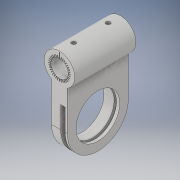
# Autodesk Inventor part: cam_holder_wrist_part
Saved by Autodesk Inventor 2019 (Build 230136000, 136)
## iProperties
Created: 2024-08-06
Part Number: cam_holder_wrist_part
Material: Generisch
Document SubType Name: Modeling
Designer: nic
Density: 1 g/cm^3
Appearance: Vorgabe
Author: nic
Autodesk Inventor part; units mm, degrees
ref_plane "YZ Plane" through (0, 0, 0) normal (1, 0, 0) x (0, 1, 0)
ref_plane "XY Plane" through (0, 0, 0) normal (0, 0, 1) x (1, 0, 0)
sketch "Skizze1" plane through (0, 0, 0) normal (1, 0, 0) x (0, 1, 0)
  line L0 (0, 0) -> (0, 35) construction
  circle A0 centre (0, 35) radius 35
  circle A1 centre (0, 35) radius 25.05
  dimension "d0" = 35
  dimension "d1" = 50.1
  constraints: 2 coincident, 2 end point, 1 centre point, 1 vertical, 1 vertical alignment, 2 other
  measures "d0" distance of L0.start L0.end
  measures "d1" diameter of A1
extrude "Extrusion1" add sketch "Skizze1" along normal blind 18
sketch "Skizze2" plane through (0, 0, 0) normal (0, 0, 1) x (1, 0, 0)
  line L0 (18, -35) -> (18, 35) construction
  line L1 (0, 35) -> (0, -35) construction
  line L2 (0, 35) -> (18, 35) projected
  line L3 (9, 35) -> (9, 60) construction
  circle A0 centre (9, 60) radius 10.05
  circle A1 centre (9, 60) radius 17.5
  point P0 (0, 0)
  dimension "d5" = 25
  dimension "d6" = 20.1
  dimension "d7" = 35
  constraints: 2 centre point, 2 coincident, 2 end point, 1 midpoint, 1 vertical
  measures "d5" distance of L3.start L3.end
  measures "d6" diameter of A0
  measures "d7" diameter of A1
extrude "Extrusion2" add sketch "Skizze2" along normal blind 70
sketch "Skizze3" plane through (0, 0, 0) normal (0, 0, 1) x (1, 0, 0)
  line L0 (18, -35) -> (18, 35) construction
  line L1 (0, 35) -> (0, -35) construction
  circle A0 centre (9, 60) radius 17.5 construction
  line L2 (18, -35) -> (18, 35) projected
  line L3 (18, 0) -> (0, 0)
  line L4 (0, 0) -> (0, 44.9917)
  line L5 (18, 44.9917) -> (18, 0)
  arc A1 (0, 44.9917) -> (18, 44.9917) centre (9, 60) ccw
  point P0 (0, 0)
  constraints: 6 end point, 2 point on circle, 1 centre point, 1 coincident, 1 horizontal, 1 midpoint, 1 parallel, 1 perpendicular, 2 other
extrude "Extrusion3" add sketch "Skizze3" along normal blind 70
sketch "Skizze4" plane through (0, 0, 0) normal (-1, 0, 0) x (0, 0, 1)
  line L0 (9.95, 0) -> (60.05, 0) projected
  circle A0 centre (35, 0) radius 25.05
  point P0 (0, 0)
  constraints: 1 centre point, 1 midpoint
extrude "Extrusion4" cut sketch "Skizze4" against normal through all
ref_plane "Arbeitsebene1" through (13, 0, 0) normal (1, 0, 0) x (0, 0, -1)
sketch "Skizze5" plane through (13, 0, 0) normal (1, 0, 0) x (0, 0, -1)
  circle A0 centre (-35, 0) radius 25.05 construction
  arc A1 (-70, 0) -> (0, 0) centre (-35, 0) ccw construction
  line L0 (0, 44.9917) -> (0, 0) construction
  line L1 (-70, 44.9917) -> (0, 44.9917) construction
  line L2 (-70, 0) -> (-70, 44.9917) construction
  circle A2 centre (-35, 0) radius 25.05
  arc A3 (-59.4438, 25.05) -> (-10.5562, 25.05) centre (-35, 0) ccw
  line L3 (-70, 0) -> (-70, 44.9917) projected
  line L4 (-70, 25.05) -> (0, 25.05)
  line L5 (0, 25.05) -> (0, 0)
  line L6 (-70, 0) -> (-70, 25.05)
  constraints: 6 end point, 4 point on circle, 3 point on line, 2 centre point, 2 coincident, 1 horizontal, 1 parallel, 1 perpendicular
extrude "Extrusion5" cut sketch "Skizze5" against normal blind 1.325 and the other way blind 1.325
sketch "Skizze6" plane through (13, 0, 0) normal (1, 0, 0) x (0, 0, -1)
  circle A0 centre (-35, 0) radius 25.05 construction
  arc A1 (-70, 0) -> (0, 0) centre (-35, 0) ccw construction
  line L0 (0, 44.9917) -> (0, 0) construction
  line L1 (-70, 44.9917) -> (0, 44.9917) construction
  line L2 (-70, 0) -> (-70, 44.9917) construction
  arc A2 (-70, 0) -> (0, 0) centre (-35, 0) ccw projected
  line L3 (-70, 25.05) -> (-70, 0) projected
  line L4 (0, 0) -> (0, 25.05) projected
  line L5 (-70, 25.05) -> (-35, 25.05) projected
  line L6 (-35, 25.05) -> (0, 25.05) projected
  line L7 (-65, 39.9917) -> (-5, 39.9917)
  line L8 (-5, 39.9917) -> (-5, 0)
  arc A3 (-65, 0) -> (-5, 0) centre (-35, 0) ccw
  line L9 (-65, 0) -> (-65, 39.9917)
  line L10 (-65, 25.05) -> (-5, 25.05)
  dimension "d19" = 5
  constraints: 8 end point, 4 point on line, 2 point on circle, 1 centre point, 1 vertical alignment, 3 other
  measures "d19" distance between parallel lines of L2 L9
extrude "Extrusion6" cut sketch "Skizze6" against normal blind 2.5 and the other way blind 2.5 contours L3 L5 L9 A3 L8 L6 L4 A2
ref_plane "Arbeitsebene2" through (0, 78, 0) normal (0, 1, 0) x (-1, 0, 0)
sketch "Skizze7" plane through (0, 78, 0) normal (0, 1, 0) x (-1, 0, 0)
  line L0 (-19.05, 70) -> (1.05, 70) projected
  line L1 (-9, 70) -> (-9, 0)
  point P0 (0, 0)
  point P1 (-9, 53.6501)
  point P2 (-9, 14.2598)
  constraints: 2 end point, 2 point on line, 1 midpoint, 1 vertical
hole "Bohrung1" at (9, 78, 53.6501) at (9, 78, 14.2598) direction (0, -1, 0) diameter 3.8 depth 10 tip angle 118 counterbore diameter 5 counterbore depth 2
sketch "Skizze8" plane through (0, 0, 70) normal (0, 0, 1) x (1, 0, 0)
  circle A0 centre (9, 60) radius 10.05 construction
  arc A1 (18, 44.9917) -> (0, 44.9917) centre (9, 60) ccw construction
  line L0 (8.75, 67.55) -> (9.25, 67.55)
  line L1 (9.25, 67.55) -> (9.25, 72.55)
  line L2 (9.25, 72.55) -> (8.75, 72.55)
  line L3 (8.75, 72.55) -> (8.75, 67.55)
  line L4 (8.75, 67.55) -> (9.25, 72.55) construction
  line L5 (9.25, 67.55) -> (8.75, 72.55) construction
  line L6 (7.4428, 67.3919) -> (7.9352, 67.4787)
  line L7 (7.9352, 67.4787) -> (7.0669, 72.4027)
  line L8 (7.0669, 72.4027) -> (6.5745, 72.3159)
  line L9 (6.5745, 72.3159) -> (7.4428, 67.3919)
  line L10 (7.4428, 67.3919) -> (7.0669, 72.4027) construction
  line L11 (7.9352, 67.4787) -> (6.5745, 72.3159) construction
  line L12 (6.1828, 67.0092) -> (6.6527, 67.1802)
  line L13 (6.6527, 67.1802) -> (4.9426, 71.8786)
  line L14 (4.9426, 71.8786) -> (4.4727, 71.7076)
  line L15 (4.4727, 71.7076) -> (6.1828, 67.0092)
  line L16 (6.1828, 67.0092) -> (4.9426, 71.8786) construction
  line L17 (6.6527, 67.1802) -> (4.4727, 71.7076) construction
  line L18 (5.0085, 66.4135) -> (5.4415, 66.6635)
  line L19 (5.4415, 66.6635) -> (2.9415, 70.9936)
  line L20 (2.9415, 70.9936) -> (2.5085, 70.7436)
  line L21 (2.5085, 70.7436) -> (5.0085, 66.4135)
  line L22 (5.0085, 66.4135) -> (2.9415, 70.9936) construction
  line L23 (5.4415, 66.6635) -> (2.5085, 70.7436) construction
  line L24 (3.9554, 65.6229) -> (4.3385, 65.9443)
  line L25 (4.3385, 65.9443) -> (1.1245, 69.7746)
  line L26 (1.1245, 69.7746) -> (0.7415, 69.4532)
  line L27 (0.7415, 69.4532) -> (3.9554, 65.6229)
  line L28 (3.9554, 65.6229) -> (1.1245, 69.7746) construction
  line L29 (4.3385, 65.9443) -> (0.7415, 69.4532) construction
  line L30 (3.0557, 64.6615) -> (3.3771, 65.0446)
  line L31 (3.3771, 65.0446) -> (-0.4532, 68.2585)
  line L32 (-0.4532, 68.2585) -> (-0.7746, 67.8755)
  line L33 (-0.7746, 67.8755) -> (3.0557, 64.6615)
  line L34 (3.0557, 64.6615) -> (-0.4532, 68.2585) construction
  line L35 (3.3771, 65.0446) -> (-0.7746, 67.8755) construction
  line L36 (2.3365, 63.5585) -> (2.5865, 63.9915)
  line L37 (2.5865, 63.9915) -> (-1.7436, 66.4915)
  line L38 (-1.7436, 66.4915) -> (-1.9936, 66.0585)
  line L39 (-1.9936, 66.0585) -> (2.3365, 63.5585)
  line L40 (2.3365, 63.5585) -> (-1.7436, 66.4915) construction
  line L41 (2.5865, 63.9915) -> (-1.9936, 66.0585) construction
  line L42 (1.8198, 62.3473) -> (1.9908, 62.8172)
  line L43 (1.9908, 62.8172) -> (-2.7076, 64.5273)
  line L44 (-2.7076, 64.5273) -> (-2.8786, 64.0574)
  line L45 (-2.8786, 64.0574) -> (1.8198, 62.3473)
  line L46 (1.8198, 62.3473) -> (-2.7076, 64.5273) construction
  line L47 (1.9908, 62.8172) -> (-2.8786, 64.0574) construction
  line L48 (1.5213, 61.0648) -> (1.6081, 61.5572)
  line L49 (1.6081, 61.5572) -> (-3.3159, 62.4255)
  line L50 (-3.3159, 62.4255) -> (-3.4027, 61.9331)
  line L51 (-3.4027, 61.9331) -> (1.5213, 61.0648)
  line L52 (1.5213, 61.0648) -> (-3.3159, 62.4255) construction
  line L53 (1.6081, 61.5572) -> (-3.4027, 61.9331) construction
  line L54 (1.45, 59.75) -> (1.45, 60.25)
  line L55 (1.45, 60.25) -> (-3.55, 60.25)
  line L56 (-3.55, 60.25) -> (-3.55, 59.75)
  line L57 (-3.55, 59.75) -> (1.45, 59.75)
  line L58 (1.45, 59.75) -> (-3.55, 60.25) construction
  line L59 (1.45, 60.25) -> (-3.55, 59.75) construction
  line L60 (1.6081, 58.4428) -> (1.5213, 58.9352)
  line L61 (1.5213, 58.9352) -> (-3.4027, 58.0669)
  line L62 (-3.4027, 58.0669) -> (-3.3159, 57.5745)
  line L63 (-3.3159, 57.5745) -> (1.6081, 58.4428)
  line L64 (1.6081, 58.4428) -> (-3.4027, 58.0669) construction
  line L65 (1.5213, 58.9352) -> (-3.3159, 57.5745) construction
  line L66 (1.9908, 57.1828) -> (1.8198, 57.6527)
  line L67 (1.8198, 57.6527) -> (-2.8786, 55.9426)
  line L68 (-2.8786, 55.9426) -> (-2.7076, 55.4727)
  line L69 (-2.7076, 55.4727) -> (1.9908, 57.1828)
  line L70 (1.9908, 57.1828) -> (-2.8786, 55.9426) construction
  line L71 (1.8198, 57.6527) -> (-2.7076, 55.4727) construction
  line L72 (2.5865, 56.0085) -> (2.3365, 56.4415)
  line L73 (2.3365, 56.4415) -> (-1.9936, 53.9415)
  line L74 (-1.9936, 53.9415) -> (-1.7436, 53.5085)
  line L75 (-1.7436, 53.5085) -> (2.5865, 56.0085)
  line L76 (2.5865, 56.0085) -> (-1.9936, 53.9415) construction
  line L77 (2.3365, 56.4415) -> (-1.7436, 53.5085) construction
  line L78 (3.3771, 54.9554) -> (3.0557, 55.3385)
  line L79 (3.0557, 55.3385) -> (-0.7746, 52.1245)
  line L80 (-0.7746, 52.1245) -> (-0.4532, 51.7415)
  line L81 (-0.4532, 51.7415) -> (3.3771, 54.9554)
  line L82 (3.3771, 54.9554) -> (-0.7746, 52.1245) construction
  line L83 (3.0557, 55.3385) -> (-0.4532, 51.7415) construction
  line L84 (4.3385, 54.0557) -> (3.9554, 54.3771)
  line L85 (3.9554, 54.3771) -> (0.7415, 50.5468)
  line L86 (0.7415, 50.5468) -> (1.1245, 50.2254)
  line L87 (1.1245, 50.2254) -> (4.3385, 54.0557)
  line L88 (4.3385, 54.0557) -> (0.7415, 50.5468) construction
  line L89 (3.9554, 54.3771) -> (1.1245, 50.2254) construction
  line L90 (5.4415, 53.3365) -> (5.0085, 53.5865)
  line L91 (5.0085, 53.5865) -> (2.5085, 49.2564)
  line L92 (2.5085, 49.2564) -> (2.9415, 49.0064)
  line L93 (2.9415, 49.0064) -> (5.4415, 53.3365)
  line L94 (5.4415, 53.3365) -> (2.5085, 49.2564) construction
  line L95 (5.0085, 53.5865) -> (2.9415, 49.0064) construction
  line L96 (6.6527, 52.8198) -> (6.1828, 52.9908)
  line L97 (6.1828, 52.9908) -> (4.4727, 48.2924)
  line L98 (4.4727, 48.2924) -> (4.9426, 48.1214)
  line L99 (4.9426, 48.1214) -> (6.6527, 52.8198)
  line L100 (6.6527, 52.8198) -> (4.4727, 48.2924) construction
  line L101 (6.1828, 52.9908) -> (4.9426, 48.1214) construction
  line L102 (7.9352, 52.5213) -> (7.4428, 52.6081)
  line L103 (7.4428, 52.6081) -> (6.5745, 47.6841)
  line L104 (6.5745, 47.6841) -> (7.0669, 47.5973)
  line L105 (7.0669, 47.5973) -> (7.9352, 52.5213)
  line L106 (7.9352, 52.5213) -> (6.5745, 47.6841) construction
  line L107 (7.4428, 52.6081) -> (7.0669, 47.5973) construction
  line L108 (9.25, 52.45) -> (8.75, 52.45)
  line L109 (8.75, 52.45) -> (8.75, 47.45)
  line L110 (8.75, 47.45) -> (9.25, 47.45)
  line L111 (9.25, 47.45) -> (9.25, 52.45)
  line L112 (9.25, 52.45) -> (8.75, 47.45) construction
  line L113 (8.75, 52.45) -> (9.25, 47.45) construction
  line L114 (10.5572, 52.6081) -> (10.0648, 52.5213)
  line L115 (10.0648, 52.5213) -> (10.9331, 47.5973)
  line L116 (10.9331, 47.5973) -> (11.4255, 47.6841)
  line L117 (11.4255, 47.6841) -> (10.5572, 52.6081)
  line L118 (10.5572, 52.6081) -> (10.9331, 47.5973) construction
  line L119 (10.0648, 52.5213) -> (11.4255, 47.6841) construction
  line L120 (11.8172, 52.9908) -> (11.3473, 52.8198)
  line L121 (11.3473, 52.8198) -> (13.0574, 48.1214)
  line L122 (13.0574, 48.1214) -> (13.5273, 48.2924)
  line L123 (13.5273, 48.2924) -> (11.8172, 52.9908)
  line L124 (11.8172, 52.9908) -> (13.0574, 48.1214) construction
  line L125 (11.3473, 52.8198) -> (13.5273, 48.2924) construction
  line L126 (12.9915, 53.5865) -> (12.5585, 53.3365)
  line L127 (12.5585, 53.3365) -> (15.0585, 49.0064)
  line L128 (15.0585, 49.0064) -> (15.4915, 49.2564)
  line L129 (15.4915, 49.2564) -> (12.9915, 53.5865)
  line L130 (12.9915, 53.5865) -> (15.0585, 49.0064) construction
  line L131 (12.5585, 53.3365) -> (15.4915, 49.2564) construction
  line L132 (14.0446, 54.3771) -> (13.6615, 54.0557)
  line L133 (13.6615, 54.0557) -> (16.8755, 50.2254)
  line L134 (16.8755, 50.2254) -> (17.2585, 50.5468)
  line L135 (17.2585, 50.5468) -> (14.0446, 54.3771)
  line L136 (14.0446, 54.3771) -> (16.8755, 50.2254) construction
  line L137 (13.6615, 54.0557) -> (17.2585, 50.5468) construction
  line L138 (14.9443, 55.3385) -> (14.6229, 54.9554)
  line L139 (14.6229, 54.9554) -> (18.4532, 51.7415)
  line L140 (18.4532, 51.7415) -> (18.7746, 52.1245)
  line L141 (18.7746, 52.1245) -> (14.9443, 55.3385)
  line L142 (14.9443, 55.3385) -> (18.4532, 51.7415) construction
  line L143 (14.6229, 54.9554) -> (18.7746, 52.1245) construction
  line L144 (15.6635, 56.4415) -> (15.4135, 56.0085)
  line L145 (15.4135, 56.0085) -> (19.7436, 53.5085)
  line L146 (19.7436, 53.5085) -> (19.9936, 53.9415)
  line L147 (19.9936, 53.9415) -> (15.6635, 56.4415)
  line L148 (15.6635, 56.4415) -> (19.7436, 53.5085) construction
  line L149 (15.4135, 56.0085) -> (19.9936, 53.9415) construction
  line L150 (16.1802, 57.6527) -> (16.0092, 57.1828)
  line L151 (16.0092, 57.1828) -> (20.7076, 55.4727)
  line L152 (20.7076, 55.4727) -> (20.8786, 55.9426)
  line L153 (20.8786, 55.9426) -> (16.1802, 57.6527)
  line L154 (16.1802, 57.6527) -> (20.7076, 55.4727) construction
  line L155 (16.0092, 57.1828) -> (20.8786, 55.9426) construction
  line L156 (16.4787, 58.9352) -> (16.3919, 58.4428)
  line L157 (16.3919, 58.4428) -> (21.3159, 57.5745)
  line L158 (21.3159, 57.5745) -> (21.4027, 58.0669)
  line L159 (21.4027, 58.0669) -> (16.4787, 58.9352)
  line L160 (16.4787, 58.9352) -> (21.3159, 57.5745) construction
  line L161 (16.3919, 58.4428) -> (21.4027, 58.0669) construction
  line L162 (16.55, 60.25) -> (16.55, 59.75)
  line L163 (16.55, 59.75) -> (21.55, 59.75)
  line L164 (21.55, 59.75) -> (21.55, 60.25)
  line L165 (21.55, 60.25) -> (16.55, 60.25)
  line L166 (16.55, 60.25) -> (21.55, 59.75) construction
  line L167 (16.55, 59.75) -> (21.55, 60.25) construction
  line L168 (16.3919, 61.5572) -> (16.4787, 61.0648)
  line L169 (16.4787, 61.0648) -> (21.4027, 61.9331)
  line L170 (21.4027, 61.9331) -> (21.3159, 62.4255)
  line L171 (21.3159, 62.4255) -> (16.3919, 61.5572)
  line L172 (16.3919, 61.5572) -> (21.4027, 61.9331) construction
  line L173 (16.4787, 61.0648) -> (21.3159, 62.4255) construction
  line L174 (16.0092, 62.8172) -> (16.1802, 62.3473)
  line L175 (16.1802, 62.3473) -> (20.8786, 64.0574)
  line L176 (20.8786, 64.0574) -> (20.7076, 64.5273)
  line L177 (20.7076, 64.5273) -> (16.0092, 62.8172)
  line L178 (16.0092, 62.8172) -> (20.8786, 64.0574) construction
  line L179 (16.1802, 62.3473) -> (20.7076, 64.5273) construction
  line L180 (15.4135, 63.9915) -> (15.6635, 63.5585)
  line L181 (15.6635, 63.5585) -> (19.9936, 66.0585)
  line L182 (19.9936, 66.0585) -> (19.7436, 66.4915)
  line L183 (19.7436, 66.4915) -> (15.4135, 63.9915)
  line L184 (15.4135, 63.9915) -> (19.9936, 66.0585) construction
  line L185 (15.6635, 63.5585) -> (19.7436, 66.4915) construction
  line L186 (14.6229, 65.0446) -> (14.9443, 64.6615)
  line L187 (14.9443, 64.6615) -> (18.7746, 67.8755)
  line L188 (18.7746, 67.8755) -> (18.4532, 68.2585)
  line L189 (18.4532, 68.2585) -> (14.6229, 65.0446)
  line L190 (14.6229, 65.0446) -> (18.7746, 67.8755) construction
  line L191 (14.9443, 64.6615) -> (18.4532, 68.2585) construction
  line L192 (13.6615, 65.9443) -> (14.0446, 65.6229)
  line L193 (14.0446, 65.6229) -> (17.2585, 69.4532)
  line L194 (17.2585, 69.4532) -> (16.8755, 69.7746)
  line L195 (16.8755, 69.7746) -> (13.6615, 65.9443)
  line L196 (13.6615, 65.9443) -> (17.2585, 69.4532) construction
  line L197 (14.0446, 65.6229) -> (16.8755, 69.7746) construction
  line L198 (12.5585, 66.6635) -> (12.9915, 66.4135)
  line L199 (12.9915, 66.4135) -> (15.4915, 70.7436)
  line L200 (15.4915, 70.7436) -> (15.0585, 70.9936)
  line L201 (15.0585, 70.9936) -> (12.5585, 66.6635)
  line L202 (12.5585, 66.6635) -> (15.4915, 70.7436) construction
  line L203 (12.9915, 66.4135) -> (15.0585, 70.9936) construction
  line L204 (11.3473, 67.1802) -> (11.8172, 67.0092)
  line L205 (11.8172, 67.0092) -> (13.5273, 71.7076)
  line L206 (13.5273, 71.7076) -> (13.0574, 71.8786)
  line L207 (13.0574, 71.8786) -> (11.3473, 67.1802)
  line L208 (11.3473, 67.1802) -> (13.5273, 71.7076) construction
  line L209 (11.8172, 67.0092) -> (13.0574, 71.8786) construction
  line L210 (10.0648, 67.4787) -> (10.5572, 67.3919)
  line L211 (10.5572, 67.3919) -> (11.4255, 72.3159)
  line L212 (11.4255, 72.3159) -> (10.9331, 72.4027)
  line L213 (10.9331, 72.4027) -> (10.0648, 67.4787)
  line L214 (10.0648, 67.4787) -> (11.4255, 72.3159) construction
  line L215 (10.5572, 67.3919) -> (10.9331, 72.4027) construction
  point P0 (0, 0)
  point P1 (9, 70.05)
  point P2 (7.2548, 69.8973)
  point P3 (5.5627, 69.4439)
  point P4 (3.975, 68.7036)
  point P5 (2.54, 67.6987)
  point P6 (1.3013, 66.46)
  point P7 (0.2964, 65.025)
  point P8 (-0.4439, 63.4373)
  point P9 (-0.8973, 61.7452)
  point P10 (-1.05, 60)
  point P11 (-0.8973, 58.2548)
  point P12 (-0.4439, 56.5627)
  point P13 (0.2964, 54.975)
  point P14 (1.3013, 53.54)
  point P15 (2.54, 52.3013)
  point P16 (3.975, 51.2964)
  point P17 (5.5627, 50.5561)
  point P18 (7.2548, 50.1027)
  point P19 (9, 49.95)
  point P20 (10.7452, 50.1027)
  point P21 (12.4373, 50.5561)
  point P22 (14.025, 51.2964)
  point P23 (15.46, 52.3013)
  point P24 (16.6987, 53.54)
  point P25 (17.7036, 54.975)
  point P26 (18.4439, 56.5627)
  point P27 (18.8973, 58.2548)
  point P28 (19.05, 60)
  point P29 (18.8973, 61.7452)
  point P30 (18.4439, 63.4373)
  point P31 (17.7036, 65.025)
  point P32 (16.6987, 66.46)
  point P33 (15.46, 67.6987)
  point P34 (14.025, 68.7036)
  point P35 (12.4373, 69.4439)
  point P36 (10.7452, 69.8973)
  dimension "d32" = 0.5
  dimension "d33" = 5
  dimension "d36" = 360
  constraints: 432 end point, 72 midpoint, 2 parallel, 1 horizontal, 1 perpendicular, 1 vertical alignment, 398 other
  measures "d32" distance of L2.end L1.end
  measures "d33" distance of L1.end L0.end
extrude "Extrusion7" cut sketch "Skizze8" against normal blind 0.5
sketch "Skizze9" plane through (0, 0, 70) normal (0, 0, 1) x (1, 0, 0)
  line L0 (9.25, 72.55) -> (9.25, 70.0469) projected
  line L1 (8.75, 70.0469) -> (8.75, 72.55) projected
  line L2 (8.75, 72.55) -> (9.25, 72.55) projected
  line L3 (11.5, 76) -> (6.5, 76) projected
  line L4 (8.75, 69.1) -> (9.25, 69.1)
  line L5 (9.25, 69.1) -> (9.25, 76)
  line L6 (9.25, 76) -> (8.75, 76)
  line L7 (8.75, 76) -> (8.75, 69.1)
  line L8 (8.75, 69.1) -> (9.25, 76) construction
  line L9 (9.25, 69.1) -> (8.75, 76) construction
  point P0 (0, 0)
  point P1 (9, 72.55)
  constraints: 12 end point, 3 midpoint, 2 parallel, 1 horizontal, 1 perpendicular, 1 point on line
extrude "Extrusion8" cut sketch "Skizze9" against normal blind 0.5
